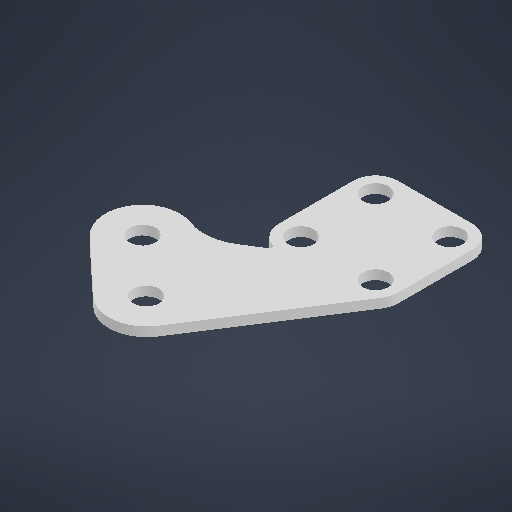
# Autodesk Inventor part: lbMountInside
Saved by Autodesk Inventor 2025.2 (Build 292293000, 293)
## iProperties
Created: 2025-03-24
Part Number: lbMountInside
Material: Generic
Document SubType Name: Modeling
Designer: Jahan
Density: 1 g/cm^3
Appearance: Default
Author: Jahan
Autodesk Inventor part; units mm, degrees
ref_plane "YZ Plane" through (0, 0, 0) normal (1, 0, 0) x (0, 1, 0)
ref_plane "XZ Plane" through (0, 0, 0) normal (0, 1, 0) x (-1, 0, 0)
ref_plane "XY Plane" through (0, 0, 0) normal (0, 0, 1) x (1, 0, 0)
sketch "Sketch1" plane through (0, 0, 0) normal (0, 1, 0) x (-1, 0, 0)
  ellipse E0 centre (13.1478, 12.5921) end of major axis (11.6568, 10.9957) minor radius 2.1844
  ellipse E1 centre (3.8663, 21.2606) end of major axis (2.3753, 19.6642) minor radius 2.1844
  circle A0 centre (-0.5698, -0.6484) radius 2.1844
  circle A1 centre (-0.5698, -13.3484) radius 2.1844
  circle A2 centre (-13.2698, -13.3484) radius 2.1844
  circle A3 centre (-13.2698, -0.6484) radius 2.1844
  line L0 (8.2005, 25.9014) -> (17.4821, 17.2329)
  line L1 (-1.4719, 24.6996) -> (-16.4726, 1.415)
  line L2 (-17.0798, -0.6484) -> (-17.0798, -13.3493)
  line L3 (-13.2698, -17.1584) -> (-0.5698, -17.1584)
  line L4 (3.2402, -13.3484) -> (3.2402, -0.6484)
  arc A4 (10.9525, 6.6337) -> (3.8547, 5.9108) centre (8.1433, -0.991) ccw
  arc A5 (10.9525, 6.6337) -> (17.4821, 17.2329) centre (13.1478, 12.5921) ccw
  arc A6 (8.2005, 25.9014) -> (-1.4719, 24.6996) centre (3.8663, 21.2606) ccw
  arc A7 (0.5589, 3.8629) -> (0.662, 2.957) centre (0.8251, 3.4344) ccw
  line L5 (3.8547, 5.9108) -> (0.5589, 3.8629)
  arc A8 (3.2402, -0.6484) -> (0.662, 2.957) centre (-0.5698, -0.6484) ccw
  arc A9 (-0.5698, -17.1584) -> (3.2402, -13.3484) centre (-0.5698, -13.3484) ccw
  arc A10 (-16.4726, 1.415) -> (-17.0798, -0.6484) centre (-13.2698, -0.6484) ccw
  arc A11 (-17.0798, -13.3493) -> (-13.2698, -17.1584) centre (-13.2698, -13.3484) ccw
  point P0 (0, 0)
  constraints: 16 point on circle, 12 centre point, 12 end point, 5 coincident, 1 tangent, 1 vertical, 6 other
extrude "Extrusion1" add sketch "Sketch1" along normal blind 1.5875
body "Solid1"
